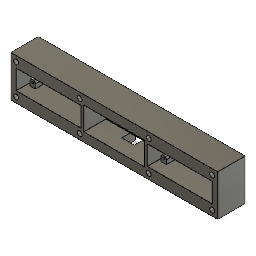
Bracket-v1.1-FusionProject (Autodesk Fusion 360 design; units mm, degrees)
Autodesk Fusion 360 part; units mm, degrees
note: some values were not read from the file. Set by a fixed rule: which sketch regions a step uses.
sketch "Sketch1" plane through (0, 0, 0) normal (0, 0, 1) x (1, 0, 0)
  line L0 (-70, -6.0833) -> (-25, -6.0833)
  line L1 (-25, -6.0833) -> (-25, 6.0667)
  line L2 (-25, 6.0667) -> (-70, 6.0667)
  line L3 (-70, 6.0667) -> (-70, -6.0833)
  circle A0 centre (-27.9, 3.9667) radius 0.925
  line L4 (-70, -0.0083) -> (-25, -0.0083)
  line L5 (-47.5, 6.0667) -> (-47.5, -6.0833)
  circle A1 centre (-67.1, -3.9833) radius 0.925
  line L6 (16.5, 7.375) -> (-16.5, 7.375)
  line L7 (-16.5, -7.375) -> (16.5, -7.375)
  line L8 (16.5, -7.375) -> (16.5, 7.375)
  line L9 (19, 0) -> (21, 0)
  line L10 (16.5, 0) -> (19, 0)
  circle A2 centre (17.875, 0) radius 3.125
  circle A3 centre (17.875, 0) radius 1.125
  line L11 (-16.5, 7.375) -> (-16.5, -7.375)
  line L12 (3.5, -12.375) -> (-3.5, -7.375) construction
  line L13 (-19, 0) -> (-21, 0)
  line L14 (0, 7.375) -> (0, -12.375)
  line L15 (3.5, -7.375) -> (3.5, -12.375)
  line L16 (-3.5, -12.375) -> (3.5, -7.375) construction
  circle A4 centre (-17.875, 0) radius 3.125
  circle A5 centre (-17.875, 0) radius 1.125
  line L17 (-16.5, 0) -> (16.5, 0)
  line L18 (-16.5, 0) -> (-19, 0)
  line L19 (3.5, -12.375) -> (-3.5, -12.375)
  line L20 (-3.5, -7.375) -> (3.5, -7.375)
  line L21 (-3.5, -12.375) -> (-3.5, -7.375)
  line L22 (75, 15) -> (-75, 15)
  line L23 (-75, 15) -> (-75, -15)
  line L24 (-75, -15) -> (75, -15)
  line L25 (75, -15) -> (75, 15)
  line L26 (75, 15) -> (-75, -15) construction
  line L27 (-75, 15) -> (75, -15) construction
  line L28 (-24, 7.0667) -> (-71, 7.0667)
  line L29 (-71, 7.0667) -> (-71, -7.0833)
  line L30 (-71, -7.0833) -> (-24, -7.0833)
  line L31 (-24, -7.0833) -> (-24, 7.0667)
  line L32 (-4.5, -6.375) -> (4.5, -6.375)
  line L33 (4.5, -6.375) -> (4.5, -13.375)
  line L34 (4.5, -13.375) -> (-4.5, -13.375)
  line L35 (-4.5, -13.375) -> (-4.5, -6.375)
  line L36 (-21, 0) -> (-22, 0)
  line L37 (-17.5, -8.375) -> (17.5, -8.375)
  line L38 (17.5, -8.375) -> (17.5, 8.375)
  line L39 (17.5, 8.375) -> (-17.5, 8.375)
  line L40 (-17.5, 8.375) -> (-17.5, -8.375)
  line L41 (-22, 7.375) -> (-22, 0)
  line L42 (-17.5, -8.375) -> (-22, -8.375)
  line L43 (-22, -8.375) -> (-22, 0)
  line L44 (-17.5, 8.375) -> (-22, 8.375)
  line L45 (-22, 8.375) -> (-22, 7.375)
  line L46 (21, 0) -> (22, 0)
  line L47 (22, 0) -> (22, 8.375)
  line L48 (22, 8.375) -> (17.5, 8.375)
  line L49 (22, 0) -> (22, -8.375)
  line L50 (22, -8.375) -> (17.5, -8.375)
  circle A6 centre (-67.1, -3.9833) radius 0.675
  circle A7 centre (-27.9, 3.9667) radius 0.675
  circle A8 centre (-27.9, 3.9667) radius 1.925
  circle A9 centre (-67.1, -3.9833) radius 1.925
  line L51 (12, 5.5) -> (-12, 5.5)
  line L52 (-12, 5.5) -> (-12, -5.5)
  line L53 (-12, -5.5) -> (12, -5.5)
  line L54 (12, -5.5) -> (12, 5.5)
  line L55 (12, 5.5) -> (-12, -5.5) construction
  line L56 (-12, 5.5) -> (12, -5.5) construction
  circle A10 centre (-9.2, 0) radius 1.5
  line L57 (-7.7, 0) -> (-6.7, 0)
  line L58 (-6.7, 0) -> (-6.7, -5.5)
  line L59 (-6.7, 0) -> (-6.7, 5.5)
  line L60 (-13, -6.5) -> (13, -6.5)
  line L61 (13, -6.5) -> (13, 6.5)
  line L62 (13, 6.5) -> (-13, 6.5)
  line L63 (-13, 6.5) -> (-13, -6.5)
  circle A11 centre (-71, -11) radius 1.75
  circle A12 centre (71, -11) radius 1.75
  circle A13 centre (-71, 11) radius 1.75
  circle A14 centre (71, 11) radius 1.75
  circle A15 centre (-25, 11) radius 1.75
  circle A16 centre (25, 11) radius 1.75
  circle A17 centre (-25, -11) radius 1.75
  circle A18 centre (25, -11) radius 1.75
  line L64 (-27.9, 3.9667) -> (-29.825, 3.9667)
  line L65 (-29.825, 3.9667) -> (-29.825, 7.0667)
  line L66 (-27.9, 3.9667) -> (-25.975, 3.9667)
  line L67 (-25.975, 3.9667) -> (-25.975, 7.0667)
  line L68 (-24, -7.0833) -> (-41, -7.0833)
  line L69 (-41, -7.0833) -> (-41, 1.9167)
  line L70 (-41, 1.9167) -> (-24, 1.9167)
  line L71 (-24, 1.9167) -> (-24, -7.0833)
  line L72 (-67.1, -3.9833) -> (-65.175, -3.9833)
  line L73 (-67.1, -3.9833) -> (-69.025, -3.9833)
  line L74 (-65.175, -3.9833) -> (-65.175, -7.0833)
  line L75 (-69.025, -3.9833) -> (-69.025, -7.0833)
  line L76 (25, 6.075) -> (25, -6.075)
  line L77 (25, -6.075) -> (70, -6.075)
  line L78 (70, 6.075) -> (25, 6.075)
  line L79 (71, -7.075) -> (71, 7.075)
  line L80 (24, 7.075) -> (24, -7.075)
  line L81 (24, -7.075) -> (71, -7.075)
  line L82 (71, 7.075) -> (24, 7.075)
  line L83 (25, 0) -> (70, 0)
  line L84 (47.5, 6.075) -> (47.5, -6.075)
  line L85 (71, -7.075) -> (54, -7.075)
  line L86 (54, -7.075) -> (54, 1.925)
  line L87 (71, 1.925) -> (71, -7.075)
  line L88 (54, 1.925) -> (71, 1.925)
  line L89 (25.975, -3.975) -> (25.975, -7.075)
  circle A19 centre (27.9, -3.975) radius 1.925
  circle A20 centre (27.9, -3.975) radius 0.925
  circle A21 centre (27.9, -3.975) radius 0.675
  line L90 (27.9, -3.975) -> (25.975, -3.975)
  line L91 (27.9, -3.975) -> (29.825, -3.975)
  line L92 (29.825, -3.975) -> (29.825, -7.075)
  line L93 (67.1, 3.975) -> (65.175, 3.975)
  circle A22 centre (67.1, 3.975) radius 1.925
  line L94 (65.175, 3.975) -> (65.175, 7.075)
  circle A23 centre (67.1, 3.975) radius 0.675
  circle A24 centre (67.1, 3.975) radius 0.925
  line L95 (67.1, 3.975) -> (69.025, 3.975)
  line L96 (69.025, 3.975) -> (69.025, 7.075)
  line L97 (4.5, -13.375) -> (4.5, -15)
  line L98 (-4.5, -13.375) -> (-4.5, -15)
  point P0 (-47.5, -0.0083)
  dimension "d2" = 12.15
  dimension "d5" = 1.85
  dimension "d22" = 1.85
  dimension "d47" = 2
  dimension "d48" = 2
  dimension "d49" = 33
  dimension "d51" = 2.5
  dimension "d52" = 2.5
  dimension "d53" = 2.25
  dimension "d54" = 2.25
  dimension "d55" = 7
  dimension "d56" = 5
  dimension "d57" = 150
  dimension "d58" = 30
  dimension "d63" = 1
  dimension "d83" = 24
  dimension "d84" = 11
  dimension "d85" = 3
  dimension "d87" = 1
  dimension "d93" = 3.5
  dimension "d94" = 3.5
  dimension "d96" = 3.5
  dimension "d97" = 3.5
  dimension "d98" = 3.5
  dimension "d99" = 3.5
  dimension "d100" = 3.5
  dimension "d105" = 17
  dimension "d106" = 9
  dimension "d107" = 12.15
  dimension "d108" = 1.85
  dimension "d109" = 1.85
  dimension "d110" = 17
  dimension "d111" = 9
  measures "d2" distance of L0.start L2.end
  measures "d5" diameter of A0
  measures "d22" diameter of A1
  measures "d49" distance of L7.end L7.start
  measures "d51" distance of L9.start L10.start
  measures "d52" distance of L17.start L13.start
  measures "d53" diameter of A5
  measures "d54" diameter of A3
  measures "d55" distance of L12.end L15.start
  measures "d56" distance of L16.start L12.end
  measures "d57" distance of L23.end L24.end
  measures "d58" distance of L22.end L23.end
  measures "d63" distance of L13.end L36.end
  measures "d83" distance of L52.end L53.end
  measures "d84" distance of L51.end L52.end
  measures "d85" diameter of A10
  measures "d87" distance of L57.start L57.end
  measures "d93" diameter of A11
  measures "d94" diameter of A12
  measures "d96" diameter of A14
  measures "d97" diameter of A15
  measures "d98" diameter of A16
  measures "d99" diameter of A17
  measures "d100" diameter of A18
  measures "d105" distance of L30.end L68.end
  measures "d106" distance of L30.end L70.end
  measures "d107" distance of L76.end L76.start
  measures "d108" diameter of A24
  measures "d109" diameter of A20
  measures "d110" distance of L79.start L85.end
  measures "d111" distance of L79.start L87.start
extrude "Extrude3" add sketch "Sketch1" along normal blind 20 contours L22 L23 L24 L25 L33 L35 L37 L39 L41 L42 L43 L44 L45 L47 L48 L49 L50 L97 L98 | L15 L19 L21 L33 L34 L35 L37 | L14 L15 L19 L37 | L24 L34 L97 L98 | L14 L19 L21 L37 makes body 1
extrude "Extrude4" add sketch "Sketch1" along normal blind 4 contours L0 L3 L4 L5 A9 L74 L75 | L0 L2 L3 L28 L29 L30 L65 L75 | L2 L3 L4 L5 | L0 L30 L69 L74 | L1 L2 L4 L5 A8 L65 L67 L69 L70 | L0 L4 L5 L69 | A6 L72 L73 | A6 L72 L73 | L1 L2 L28 L31 L67 L70 | A7 L64 L66 | A7 L64 L66 | L6 L8 A2 L14 L17 L61 L62 | L6 L8 A2 L11 A4 L38 L39 L40 | L6 L11 L14 A4 L17 L62 L63 | L8 L10 A2 A3 L38 | L8 A2 L17 | L14 L17 L51 L54 L61 L62 | L14 L17 L51 L52 L62 L63 | L8 L10 A2 A3 L38 | L8 A2 L17 | A2 L38 L46 L47 L48 | L9 A2 A3 L38 | L7 L8 A2 L17 L33 L60 L61 | L11 A4 L17 | L11 A4 A5 L18 L40 | L14 L17 L51 L54 | L14 L17 L51 L59 | L7 L8 A2 L33 L37 L38 | L9 A2 A3 L38 | A2 L38 L46 L49 L50 | L14 L17 L32 L33 L53 L54 L60 L61 | L11 A4 L17 | L11 A4 A5 L18 L40 | L7 L11 A4 L17 L35 L60 L63 | L13 A4 A5 L40 | A4 L36 L40 L41 L44 L45 | L14 L17 L53 L54 | L14 L17 L53 L58 | L17 L51 L52 A10 L57 L59 | L14 L17 L32 L35 L52 L53 L60 L63 | L7 L11 A4 L35 L37 L40 | L13 A4 A5 L40 | A4 L36 L40 L42 L43 | L17 L52 L53 A10 L57 L58 | L7 L15 L33 L37 | L7 L14 L20 L33 L60 | L14 L32 L33 L60 | L14 L32 L35 L60 | L17 A10 | L17 A10 | L7 L14 L20 L35 L60 | L7 L14 L15 L20 L37 | L7 L21 L35 L37 | L7 L14 L20 L21 L37 | L76 L78 L83 L84 | L76 L77 L78 L80 L81 L82 L89 L94 | L76 L77 L83 L84 L89 A19 L92 | L78 L79 L82 L83 L84 L86 L88 A22 L94 L96 | L77 L83 L84 L86 | L77 L81 L86 L92 | L93 A23 L95 | L93 A23 L95 | A21 L90 L91 | A21 L90 L91 bodies 1 makes body 2 at (-27.685, 4.6066, 1.3333) makes body 3 at (-67.4079, -4.584, 2.6667) makes body 4 at (28.115, -3.3351, 1.3333) makes body 5 at (67.3776, 4.5903, 2.6667)
extrude "Extrude5" add sketch "Sketch1" along normal blind 12 contours L0 A9 L74 L75 | L0 L30 L74 L75 | A1 A9 L72 L73 | A1 A9 L72 L73 | A1 A6 L72 L73 | A1 A6 L72 L73 | L2 L28 L65 L67 | L2 A8 L65 L67 | A0 A8 L64 L66 | A0 A8 L64 L66 | A0 A7 L64 L66 | A0 A7 L64 L66 | L78 L82 L94 L96 | L78 A22 L94 L96 | L77 L89 A19 L92 | L77 L81 L89 L92 | L93 A22 A24 L95 | L93 A22 A24 L95 | A19 A20 L90 L91 | A19 A20 L90 L91 | L93 A23 A24 L95 | L93 A23 A24 L95 | A20 A21 L90 L91 | A20 A21 L90 L91 bodies 1
extrude "Extrude6" cut sketch "Sketch1" along normal blind 2 contours L14 L17 L51 L54 L61 L62 | L14 L17 L51 L52 L62 L63 | L14 L17 L51 L54 | L14 L17 L51 L59 | L14 L17 L32 L33 L53 L54 L60 L61 | L14 L17 L53 L54 | L14 L17 L53 L58 | L17 L51 L52 A10 L57 L59 | L14 L17 L32 L35 L52 L53 L60 L63 | L17 L52 L53 A10 L57 L58 | L14 L32 L33 L60 | L14 L32 L35 L60 | L17 A10 | L17 A10 bodies 1
extrude "Extrude7" cut sketch "Sketch1" along normal blind 10 contours L15 L19 L21 L33 L34 L35 L37 | L14 L15 L19 L37 | L24 L34 L97 L98 | L14 L19 L21 L37 bodies 1
extrude "Extrude9" add sketch "Sketch1" along normal blind 10 contours L10 A3 L38 | L10 A3 L38 | L10 A3 L38 | L10 A3 L38 | A5 L18 L40 | A5 L18 L40 | A5 L18 L40 | A5 L18 L40 bodies 1
